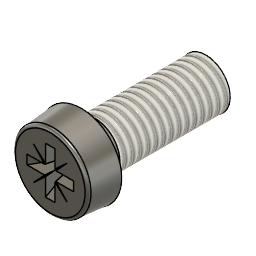
Assembly_2 (Autodesk Fusion 360 archive; units mm, degrees)
design "Cheese Head Screw BS EN ISO 7048 - M8 x 20 - Z Steel 4.6 Plain"
description: Cheese Head Screw BS EN ISO 7048 - M8 x 20 - Z
part number: BS EN ISO 7048 - Z - M8 x 20 Steel 4.6 Plain
Autodesk Fusion 360 part; units mm, degrees
sketch "Sketch1" plane through (0, 0, 0) normal (0, 1, 0) x (1, 0, 0)
  line L0 (0, -5) -> (0, 20)
  line L1 (-6.5, 0) -> (-6.0626, -5)
  line L2 (-6.5, 0) -> (-3.5625, 0)
  line L3 (0, 20) -> (-4, 20)
  line L4 (-4, 20) -> (-4, 2.5)
  line L5 (-4, 2.5) -> (-3.5625, 0.8672)
  line L6 (-3.5625, 0.8672) -> (-3.5625, 0)
  line L7 (0, -5) -> (-6.0626, -5)
  dimension "d13" = 5
  dimension "d14" = 13
  dimension "d18" = 8
  dimension "d56" = 20
  dimension "d65" = 15
  dimension "d71" = 7.125
  dimension "d77" = 2.5
  dimension "d97" = 5
  constraint vertical L0
  constraint coincident origin L0
  constraint coincident origin L2
  constraint coincident L2.end L6.end
  constraint perpendicular L0 L7
  measures "d13" angle of L0 L1
  measures "d56" distance of L2 L3
  measures "d65" angle of L5 L6
  measures "d77" distance of L2 L4.end
  measures "d97" distance of L2 L7
revolve "Revolve1" add sketch "Sketch1" angle 360 about axis through (0, 0, 5) along (0, 0, -1) makes body 1
fillet "Fillet3" radius 0.5 1 edges at (-5.6523, 2.1923, 5) on bodies 1
fillet "Fillet2" radius 0.4 1 edges at (-3.3214, 1.2883, 0) on bodies 1
sketch "Sketch2" plane through (0, 0, 5) normal (0, 0, 1) x (1, 0, 0)
  line L0 (-0.9, -0.9) -> (0.9, -0.9)
  line L1 (0.9, -0.9) -> (0.9, 0.9)
  line L2 (0.9, 0.9) -> (-0.9, 0.9)
  line L3 (-0.9, 0.9) -> (-0.9, -0.9)
  dimension "d98" = 1.8
  constraint vertical L1
  measures "d98" distance of L0 L2
extrude "Extrude2" add sketch "Sketch2" against normal blind 3.104 draft -10 separate body makes body 2
sketch "Sketch3" plane through (0, 0, 5) normal (0, 0, 1) x (1, 0, 0)
  circle A0 centre (0, 0) radius 5.6044
  line L0 (-0.75, 0.75) -> (-3.75, 0.75)
  line L1 (-3.75, 0.75) -> (-3.75, -0.75)
  line L2 (-3.75, -0.75) -> (-0.75, -0.75)
  line L3 (-0.75, -0.75) -> (-0.75, -3.75)
  line L4 (-0.75, -3.75) -> (0.75, -3.75)
  line L5 (0.75, -3.75) -> (0.75, -0.75)
  line L6 (0.75, -0.75) -> (3.75, -0.75)
  line L7 (3.75, -0.75) -> (3.75, 0.75)
  line L8 (3.75, 0.75) -> (0.75, 0.75)
  line L9 (0.75, 0.75) -> (0.75, 3.75)
  line L10 (0.75, 3.75) -> (-0.75, 3.75)
  line L11 (-0.75, 3.75) -> (-0.75, 0.75)
  dimension "d86" = 360
  dimension "d87" = 7.5
  dimension "d99" = 1.5
  constraint horizontal L0
  constraint vertical L0.start L2.end
  constraint coincident L0.start L11.end
  constraint perpendicular L7 L8
  measures "d87" distance of L4.end L10
  measures "d99" distance of L0 L2
extrude "Extrude3" add sketch "Sketch3" against normal blind 3.88 draft -4 separate body contours L0 L1 L2 L3 L4 L5 L6 L7 L8 L9 L10 L11 makes body 3
draft "Draft2" angle -30 neutral plane through (0, 0, 5) pull (0, 0, 1) 4 faces at (-0.1596, -3.6596, 3.7067) (-3.6596, 0.1596, 3.7067) (3.6596, -0.1596, 3.7067) (0.1596, 3.6596, 3.7067) on bodies 3
combine "Combine2" operation cut target body 1 tool bodies 3 2
sketch "Sketch4" plane through (0, 0, 5) normal (0, 0, 1) x (1, 0, 0)
  line L0 (0.9, 0.75) -> (3.75, 0.75)
  line L1 (0.75, 3.75) -> (0.75, 0.9)
  line L2 (0, 0) -> (2.7042, 2.7042) construction
  circle A0 centre (0, 0) radius 3.8243 construction
  line L3 (0.75, 0.9) -> (0.9, 0.75)
  line L4 (0.9, 0.75) -> (2.7042, 2.7042)
  line L5 (0.75, 0.9) -> (2.7042, 2.7042)
  line L6 (-0.9, -0.9) -> (-0.9, -0.75)
  line L7 (-0.9, 0.75) -> (-0.9, 0.9)
  line L8 (-0.9, 0.9) -> (-0.75, 0.9)
  line L9 (0.75, 0.9) -> (0.9, 0.9)
  line L10 (0.9, 0.9) -> (0.9, 0.75)
  line L11 (0.9, -0.75) -> (0.9, -0.9)
  line L12 (0.9, -0.9) -> (0.75, -0.9)
  line L13 (-0.75, -0.9) -> (-0.9, -0.9)
  point P0 (0.9, 0.9)
  constraint coincident L2.start A0.centre
  constraint coincident L1.start A0
  constraint coincident L2.end A0
  constraint coincident L1.end L3.start
  constraint coincident L0.start L3.end
  constraint coincident L2 P0
extrude "Extrude4" cut sketch "Sketch4" against normal blind 5 draft -30 bodies 1
pattern_circular "C-Pattern1" count 4 over 360 about axis through (0, 0, 1.75) along (0, 0, 1) of "Extrude4"
thread "Thread3" "ISO Metric profile 8.0 M8x1.25 M8x1.25 6g" major diameter 7.866 minor diameter 6.4455 pitch 1.25 angle 60 resizes the face on face at (-3.9801, -0.3983, -14.1667) on bodies 1
equation "adsk_nomdia = 8.00 mm"
equation "adsk_nomlen = 20.00 mm"
equation "adsk_headdia = 13.00 mm"
equation "adsk_phildia = 7.50 mm"
equation "adsk_midfillet = 0.40 mm"
equation "adsk_phildepth = 3.88 mm"
equation "adsk_shnklen = 2.50 mm"
equation "adsk_thrang = 15 deg"
equation "adsk_headang = 5 deg"
equation "d13 = adsk_headang"
equation "d14 = adsk_headdia"
equation "d18 = adsk_nomdia"
equation "adsk_philwidth = 1.50 mm"
equation "d52 = adsk_midfillet"
equation "d56 = adsk_nomlen"
equation "d65 = adsk_thrang"
equation "adsk_headh = 5.00 mm"
equation "adsk_pitch1 = 1.25 mm"
equation "adsk_shnkdia = adsk_nomdia - 0.7 * adsk_pitch1"
equation "d71 = adsk_shnkdia"
equation "adsk_headtoprad = adsk_headh * 0.1"
equation "d76 = adsk_headtoprad"
equation "d77 = adsk_shnklen"
equation "d82 = -adsk_phildepth * 0.8"
equation "d87 = adsk_phildia"
equation "d88 = -adsk_phildepth"
equation "d93 = -adsk_headh"
equation "d97 = adsk_headh"
equation "d98 = adsk_philwidth * 1.2"
equation "d99 = adsk_philwidth"
